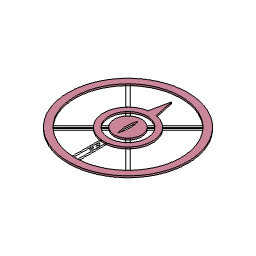
カズサ_ヘイロー_mk1 v3 (Autodesk Fusion 360 design; units mm, degrees)
Autodesk Fusion 360 part; units mm, degrees
sketch "スケッチ1" plane through (0, 0, 0) normal (0, 0, 1) x (1, 0, 0)
  circle A0 centre (0, 0) radius 110
  circle A1 centre (0, 0) radius 97.5
  circle A2 centre (0, 0) radius 25
  circle A3 centre (0, 0) radius 35
  line L0 (0, 80) -> (-7.576, 44.3577)
  line L1 (0, 0) -> (0, 110) construction
  line L2 (0, 80) -> (7.576, 44.3577)
  arc A4 (-7.576, 44.3577) -> (7.576, 44.3577) centre (0, 0) ccw
  line L3 (0, 0) -> (0, -18) construction
  line L4 (0, 0) -> (-3, 0) construction
  arc A5 (0, 18) -> (0, -18) centre (52.5, 0) ccw
  arc A6 (0, -18) -> (0, 18) centre (-52.5, 0) ccw
  line L5 (0, 0) -> (68.9429, 68.9429) construction
  line L6 (0, 0) -> (97.5, 0) construction
  line L7 (33.8703, 29.6277) -> (71.0316, 66.7889)
  line L8 (29.6277, 33.8703) -> (66.7889, 71.0316)
  line L9 (19.6712, 15.4286) -> (26.779, 22.5363)
  line L10 (15.4286, 19.6712) -> (22.5363, 26.779)
  line L11 (-33.8703, 29.6277) -> (-71.0316, 66.7889)
  line L12 (-29.6277, 33.8703) -> (-66.7889, 71.0316)
  line L13 (-19.6712, 15.4286) -> (-26.779, 22.5363)
  line L14 (-15.4286, 19.6712) -> (-22.5363, 26.779)
  line L15 (-29.6277, -33.8703) -> (-66.7889, -71.0316)
  line L16 (-33.8703, -29.6277) -> (-71.0316, -66.7889)
  line L17 (-15.4286, -19.6712) -> (-22.5363, -26.779)
  line L18 (-19.6712, -15.4286) -> (-26.779, -22.5363)
  line L19 (33.8703, -29.6277) -> (71.0316, -66.7889)
  line L20 (29.6277, -33.8703) -> (66.7889, -71.0316)
  line L21 (19.6712, -15.4286) -> (26.779, -22.5363)
  line L22 (15.4286, -19.6712) -> (22.5363, -26.779)
  line L23 (-5, -44.7214) -> (-5, -97.3717)
  line L24 (5, -44.7214) -> (5, -97.3717)
  circle A7 centre (0, -55) radius 2.6
  circle A8 centre (0, -67) radius 2.6
  point P0 (0, 18)
  point P1 (0, -18)
  dimension "d1" = 220
  dimension "d2" = 195
  dimension "d3" = 50
  dimension "d4" = 70
  dimension "d5" = 90
  dimension "d6" = 80
  dimension "d7" = 12
  dimension "d8" = 18
  dimension "d9" = 18
  dimension "d10" = 3
  dimension "d11" = 45
  dimension "d12" = 3
  dimension "d13" = 3
  dimension "d15" = 360
  dimension "d20" = 10
  dimension "d21" = 5.2
  dimension "d22" = 5.2
  dimension "d23" = 55
  dimension "d24" = 12
  dimension "d25" = 5
  dimension "d26" = 5
  constraint coincident A0.centre A1.centre
  constraint concentric A1 A2
  constraint concentric A0 A4
  constraint coincident A0 L1.end
  constraint vertical L1
  constraint coincident L0.start L1
  constraint symmetric L0.start L1 L2.start
  constraint symmetric L1 L0.end L2.end
  constraint coincident L1 P0
  constraint coincident P1 L3.end
  constraint parallel L1 L3
  constraint perpendicular L1 L4
  constraint coincident L4.end A5
  constraint coincident P0 A5.start
  constraint symmetric L1 P0 A5.start
  constraint symmetric L1 P1 L3.end
  constraint symmetric L1 A5 A6
  constraint horizontal L6
  constraint coincident A1 L5.end
  constraint coincident A1 L6.end
  constraint coincident A4 L7.start
  constraint coincident A1 L7.end
  constraint parallel L5 L7
  constraint coincident A4 L8.start
  constraint coincident A1 L8.end
  constraint symmetric L5 L7 L8
  constraint coincident A2 L9.start
  constraint coincident A3 L9.end
  constraint parallel L5 L9
  constraint coincident A2 L10.start
  constraint coincident A3 L10.end
  constraint symmetric L5 L9 L10
  constraint vertical L23
  constraint coincident A4 L23.start
  constraint coincident A1 L23.end
  constraint coincident A4 L24.start
  constraint coincident A1 L24.end
  constraint vertical L24
  constraint symmetric L3 L23 L24
  measures "d1" diameter of A0
  measures "d2" diameter of A1
  measures "d3" diameter of A2
  measures "d4" diameter of A3
  measures "d5" diameter of A4
  measures "d6" distance of A0.centre L0.start
  measures "d7" angle of L0 L1
  measures "d8" distance of A0.centre P0
  measures "d9" distance of A0.centre P1
  measures "d10" distance of A0.centre L4.end
  measures "d11" angle of L5 L6
  measures "d12" distance of L5 L7
  measures "d13" distance of L5 L9
  measures "d20" distance of L23 L24
  measures "d21" diameter of A7
  measures "d22" diameter of A8
  measures "d23" distance of A0.centre A7.centre
  measures "d24" distance of A7.centre A8.centre
  measures "d25" distance of L24 A7.centre
  measures "d26" distance of L24 A8.centre
extrude "押し出し1" add sketch "スケッチ1" along normal blind 3 contours A0 | L0 L2 A4 | A2 makes body 1 at (-61.458, 85.8309, 0) makes body 2 at (0, 56.2385, 3) makes body 3 at (10.2526, 0, 0)
extrude "押し出し2" add sketch "スケッチ1" along normal blind 3 separate body contours A1 A4 L7 L8 | A1 A4 L19 L20 | A1 A4 L11 L12 | A1 A4 L23 L24 | A1 A4 L15 L16 | A2 A3 L9 L10 | A2 A3 L21 L22 | A2 A3 L13 L14 | A2 A3 L17 L18 makes body 4 at (-18.3066, -21.6074, 0) makes body 5 at (44.4235, 43.952, 0) makes body 6 at (-43.952, 44.4235, 0) makes body 7 at (21.6074, -18.3066, 0) makes body 8 at (-21.6074, 18.3066, 0) makes body 9 at (43.952, -44.4235, 0) makes body 10 at (-44.4235, -43.952, 0) makes body 11 at (18.3066, 21.6074, 0) makes body 12 at (-0.0648, -88.1881, 0)
equation "d8 = d9"
equation "d13 = d12"
equation "d26 = d25"
